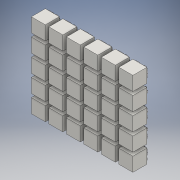
# Autodesk Inventor part: cubes&numbers
Saved by Autodesk Inventor 2017 SP1 (Build 210196100, 196)
## iProperties
Part Number: cubes&numbers
Material: Générique
Document SubType Name: Modeling
Designer: tmonglon
Density: 1 g/cm^3
Appearance: Par défaut
Author: tmonglon
Autodesk Inventor part; units mm, degrees
(part 1 of 3)
ref_plane "YZ Plane" through (0, 0, 0) normal (1, 0, 0) x (0, 1, 0)
ref_plane "XZ Plane" through (0, 0, 0) normal (0, 1, 0) x (-1, 0, 0)
ref_plane "XY Plane" through (0, 0, 0) normal (0, 0, 1) x (1, 0, 0)
sketch "Esquisse1" plane through (0, 0, 0) normal (0, 0, 1) x (1, 0, 0)
  line L0 (0, 0) -> (-8, 0)
  line L1 (-8, 0) -> (-8, 8)
  line L2 (-8, 8) -> (0, 8)
  line L3 (0, 8) -> (0, 0)
  dimension "d0" = 8
  dimension "d1" = 8
  constraints: 8 end point, 2 parallel, 1 horizontal, 1 perpendicular
  measures "d0" distance of L0.start L0.end
  measures "d1" distance of L0.end L1.end
extrude "cube" add sketch "Esquisse1" along normal blind 8
pattern_linear "Réseau rectangulaire1" count 6 spacing 10 along (1, 0, 0) count 5 spacing 10 along (0, 0, 1) of "cube"
sketch "Esquisse5" plane through (-8, 8, 40) normal (0, 1, 0) x (1, 0, 0)
  line L0 (1.5, 39) -> (6.5, 39) construction
  line L1 (6.5, 39) -> (6.5, 33) construction
  line L2 (6.5, 33) -> (1.5, 33) construction
  line L3 (1.5, 33) -> (1.5, 39) construction
  line L4 (0, 40) -> (8, 40) projected
  line L5 (0, 40) -> (0, 32) projected
  line L6 (11.5, 39) -> (16.5, 39) construction
  line L7 (16.5, 39) -> (16.5, 33) construction
  line L8 (16.5, 33) -> (11.5, 33) construction
  line L9 (11.5, 33) -> (11.5, 39) construction
  line L10 (10, 40) -> (18, 40) projected
  line L11 (10, 40) -> (10, 32) projected
  line L12 (21.5, 39) -> (26.5, 39) construction
  line L13 (26.5, 39) -> (26.5, 33) construction
  line L14 (26.5, 33) -> (21.5, 33) construction
  line L15 (21.5, 33) -> (21.5, 39) construction
  line L16 (20, 40) -> (28, 40) projected
  line L17 (20, 40) -> (20, 32) projected
  line L18 (31.5, 39) -> (36.5, 39) construction
  line L19 (36.5, 39) -> (36.5, 33) construction
  line L20 (36.5, 33) -> (31.5, 33) construction
  line L21 (31.5, 33) -> (31.5, 39) construction
  line L22 (30, 40) -> (38, 40) projected
  line L23 (30, 40) -> (30, 32) projected
  line L24 (41.5, 39) -> (46.5, 39) construction
  line L25 (46.5, 39) -> (46.5, 33) construction
  line L26 (46.5, 33) -> (41.5, 33) construction
  line L27 (41.5, 33) -> (41.5, 39) construction
  line L28 (40, 40) -> (48, 40) projected
  line L29 (40, 40) -> (40, 32) projected
  line L30 (51.5, 39) -> (56.5, 39) construction
  line L31 (56.5, 39) -> (56.5, 33) construction
  line L32 (56.5, 33) -> (51.5, 33) construction
  line L33 (51.5, 33) -> (51.5, 39) construction
  line L34 (50, 40) -> (58, 40) projected
  line L35 (50, 40) -> (50, 32) projected
  line L36 (1.5, 29) -> (6.5, 29) construction
  line L37 (6.5, 29) -> (6.5, 23) construction
  line L38 (6.5, 23) -> (1.5, 23) construction
  line L39 (1.5, 23) -> (1.5, 29) construction
  line L40 (0, 30) -> (8, 30) projected
  line L41 (0, 30) -> (0, 22) projected
  line L42 (11.5, 29) -> (16.5, 29) construction
  line L43 (16.5, 29) -> (16.5, 23) construction
  line L44 (16.5, 23) -> (11.5, 23) construction
  line L45 (11.5, 23) -> (11.5, 29) construction
  line L46 (10, 30) -> (18, 30) projected
  line L47 (10, 30) -> (10, 22) projected
  line L48 (21.5, 29) -> (26.5, 29) construction
  line L49 (26.5, 29) -> (26.5, 23) construction
  line L50 (26.5, 23) -> (21.5, 23) construction
  line L51 (21.5, 23) -> (21.5, 29) construction
  line L52 (20, 30) -> (28, 30) projected
  line L53 (20, 30) -> (20, 22) projected
  line L54 (30.5, 29) -> (37.5, 29) construction
  line L55 (37.5, 29) -> (37.5, 23) construction
  line L56 (37.5, 23) -> (30.5, 23) construction
  line L57 (30.5, 23) -> (30.5, 29) construction
  line L58 (30, 30) -> (38, 30) projected
  line L59 (30, 30) -> (30, 22) projected
  line L60 (40.5, 29) -> (47.5, 29) construction
  line L61 (47.5, 29) -> (47.5, 23) construction
  line L62 (47.5, 23) -> (40.5, 23) construction
  line L63 (40.5, 23) -> (40.5, 29) construction
  line L64 (40, 30) -> (48, 30) projected
  line L65 (40, 30) -> (40, 22) projected
  line L66 (50.5, 29) -> (57.5, 29) construction
  line L67 (57.5, 29) -> (57.5, 23) construction
  line L68 (57.5, 23) -> (50.5, 23) construction
  line L69 (50.5, 23) -> (50.5, 29) construction
  line L70 (50, 30) -> (58, 30) projected
  line L71 (50, 30) -> (50, 22) projected
  line L72 (0.5, 19) -> (7.5, 19) construction
  line L73 (7.5, 19) -> (7.5, 13) construction
  line L74 (7.5, 13) -> (0.5, 13) construction
  line L75 (0.5, 13) -> (0.5, 19) construction
  line L76 (0, 20) -> (0, 12) projected
  line L77 (0, 20) -> (8, 20) projected
  line L78 (10.5, 19) -> (17.5, 19) construction
  line L79 (17.5, 19) -> (17.5, 13) construction
  line L80 (17.5, 13) -> (10.5, 13) construction
  line L81 (10.5, 13) -> (10.5, 19) construction
  line L82 (10, 20) -> (18, 20) projected
  line L83 (18, 20) -> (18, 12) projected
  line L84 (20.5, 19) -> (27.5, 19) construction
  line L85 (27.5, 19) -> (27.5, 13) construction
  line L86 (27.5, 13) -> (20.5, 13) construction
  line L87 (20.5, 13) -> (20.5, 19) construction
  line L88 (20, 20) -> (28, 20) projected
  line L89 (28, 20) -> (28, 12) projected
  line L90 (30.5, 19) -> (37.5, 19) construction
  line L91 (37.5, 19) -> (37.5, 13) construction
  line L92 (37.5, 13) -> (30.5, 13) construction
  line L93 (30.5, 13) -> (30.5, 19) construction
  line L94 (30, 20) -> (38, 20) projected
  line L95 (30, 20) -> (30, 12) projected
  line L96 (40.5, 19) -> (47.5, 19) construction
  line L97 (47.5, 19) -> (47.5, 13) construction
  line L98 (47.5, 13) -> (40.5, 13) construction
  line L99 (40.5, 13) -> (40.5, 19) construction
  line L100 (40, 20) -> (48, 20) projected
  line L101 (40, 20) -> (40, 12) projected
  line L102 (50.5, 19) -> (57.5, 19) construction
  line L103 (57.5, 19) -> (57.5, 13) construction
  line L104 (57.5, 13) -> (50.5, 13) construction
  line L105 (50.5, 13) -> (50.5, 19) construction
  line L106 (50, 20) -> (58, 20) projected
  line L107 (58, 20) -> (58, 12) projected
  line L108 (0.5, 9) -> (7.5, 9) construction
  line L109 (7.5, 9) -> (7.5, 3) construction
  line L110 (7.5, 3) -> (0.5, 3) construction
  line L111 (0.5, 3) -> (0.5, 9) construction
  line L112 (0, 10) -> (8, 10) projected
  line L113 (8, 10) -> (8, 2) projected
  line L114 (10.5, 9) -> (17.5, 9) construction
  line L115 (17.5, 9) -> (17.5, 3) construction
  line L116 (17.5, 3) -> (10.5, 3) construction
  line L117 (10.5, 3) -> (10.5, 9) construction
  line L118 (10, 10) -> (18, 10) projected
  line L119 (18, 10) -> (18, 2) projected
  line L120 (20.5, 9) -> (27.5, 9) construction
  line L121 (27.5, 9) -> (27.5, 3) construction
  line L122 (27.5, 3) -> (20.5, 3) construction
  line L123 (20.5, 3) -> (20.5, 9) construction
  line L124 (20, 10) -> (28, 10) projected
  line L125 (28, 10) -> (28, 2) projected
  line L126 (30.5, 9) -> (37.5, 9) construction
  line L127 (37.5, 9) -> (37.5, 3) construction
  line L128 (37.5, 3) -> (30.5, 3) construction
  line L129 (30.5, 3) -> (30.5, 9) construction
  line L130 (30, 10) -> (38, 10) projected
  line L131 (38, 10) -> (38, 2) projected
  line L132 (40.5, 9) -> (47.5, 9) construction
  line L133 (47.5, 9) -> (47.5, 3) construction
  line L134 (47.5, 3) -> (40.5, 3) construction
  line L135 (40.5, 3) -> (40.5, 9) construction
  line L136 (40, 10) -> (48, 10) projected
  line L137 (48, 10) -> (48, 2) projected
  line L138 (50.5, 9) -> (57.5, 9) construction
  line L139 (57.5, 9) -> (57.5, 3) construction
  line L140 (57.5, 3) -> (50.5, 3) construction
  line L141 (50.5, 3) -> (50.5, 9) construction
  line L142 (50, 10) -> (58, 10) projected
  line L143 (50, 10) -> (50, 2) projected
  line L144 (0.5, -1) -> (7.5, -1) construction
  line L145 (7.5, -1) -> (7.5, -7) construction
  line L146 (7.5, -7) -> (0.5, -7) construction
  line L147 (0.5, -7) -> (0.5, -1) construction
  line L148 (0, 0) -> (8, 0) projected
  line L149 (0, 0) -> (0, -8) projected
  line L150 (10.5, -1) -> (17.5, -1) construction
  line L151 (17.5, -1) -> (17.5, -7) construction
  line L152 (17.5, -7) -> (10.5, -7) construction
  line L153 (10.5, -7) -> (10.5, -1) construction
  line L154 (10, 0) -> (18, 0) projected
  line L155 (18, 0) -> (18, -8) projected
  line L156 (20.5, -1) -> (27.5, -1) construction
  line L157 (27.5, -1) -> (27.5, -7) construction
  line L158 (27.5, -7) -> (20.5, -7) construction
  line L159 (20.5, -7) -> (20.5, -1) construction
  line L160 (20, 0) -> (28, 0) projected
  line L161 (20, 0) -> (20, -8) projected
  line L162 (30.5, -1) -> (37.5, -1) construction
  line L163 (37.5, -1) -> (37.5, -7) construction
  line L164 (37.5, -7) -> (30.5, -7) construction
  line L165 (30.5, -7) -> (30.5, -1) construction
  line L166 (30, 0) -> (38, 0) projected
  line L167 (30, 0) -> (30, -8) projected
  line L168 (40.5, -1) -> (47.5, -1) construction
  line L169 (47.5, -1) -> (47.5, -7) construction
  line L170 (47.5, -7) -> (40.5, -7) construction
  line L171 (40.5, -7) -> (40.5, -1) construction
  line L172 (40, 0) -> (48, 0) projected
  line L173 (48, 0) -> (48, -8) projected
  line L174 (50.5, -1) -> (57.5, -1) construction
  line L175 (57.5, -1) -> (57.5, -7) construction
  line L176 (57.5, -7) -> (50.5, -7) construction
  line L177 (50.5, -7) -> (50.5, -1) construction
  line L178 (50, 0) -> (58, 0) projected
  line L179 (50, 0) -> (50, -8) projected
  spline S0 degree 2 poles (3.7776, 35.8264) (3.7776, 35.0355) (3.5996, 33.8491) (3.4068, 33.4487) knots 0 0 0 1 2 2 2
  spline S1 degree 2 poles (3.4068, 33.4487) (3.2091, 33.0532) (2.5862, 32.6479) (2.1364, 32.6479) knots 0 0 0 1 2 2 2
  spline S2 degree 2 poles (2.1364, 32.6479) (1.6865, 32.6479) (1.0588, 33.0532) (0.861, 33.4586) knots 0 0 0 1 2 2 2
  spline S3 degree 2 poles (0.861, 33.4586) (0.6682, 33.859) (0.4903, 35.0355) (0.4903, 35.8264) knots 0 0 0 1 2 2 2
  spline S4 degree 2 poles (0.4903, 35.8264) (0.4903, 36.6371) (0.6633, 37.784) (0.866, 38.1992) knots 0 0 0 1 2 2 2
  spline S5 degree 2 poles (0.866, 38.1992) (1.0686, 38.6045) (1.6964, 39) (2.1364, 39) knots 0 0 0 1 2 2 2
  spline S6 degree 2 poles (2.1364, 39) (2.5961, 39) (3.2091, 38.5848) (3.4068, 38.1745) knots 0 0 0 1 2 2 2
  spline S7 degree 2 poles (3.4068, 38.1745) (3.6045, 37.7741) (3.7776, 36.5926) (3.7776, 35.8264) knots 0 0 0 1 2 2 2
  spline S8 degree 2 poles (2.7049, 35.8264) (2.7049, 36.9584) (2.4429, 37.8729) (2.1364, 37.8729) knots 0 0 0 1 2 2 2
  spline S9 degree 2 poles (2.1364, 37.8729) (1.825, 37.8729) (1.563, 36.9584) (1.563, 35.8215) knots 0 0 0 1 2 2 2
  spline S10 degree 2 poles (1.563, 35.8215) (1.563, 34.7043) (1.825, 33.775) (2.1364, 33.775) knots 0 0 0 1 2 2 2
  spline S11 degree 2 poles (2.1364, 33.775) (2.4429, 33.775) (2.7049, 34.7043) (2.7049, 35.8264) knots 0 0 0 1 2 2 2
  line L180 (7.3763, 32.7764) -> (4.5586, 32.7764)
  line L181 (4.5586, 32.7764) -> (4.5586, 33.8392)
  line L182 (4.5586, 33.8392) -> (5.4583, 33.8392)
  line L183 (5.4583, 33.8392) -> (5.4583, 37.0672)
  line L184 (5.4583, 37.0672) -> (4.5586, 37.0672)
  line L185 (4.5586, 37.0672) -> (4.5586, 38.0608)
  spline S12 degree 2 poles (4.5586, 38.0608) (4.7563, 38.0608) (5.1468, 38.1349) (5.2655, 38.214) knots 0 0 0 1 2 2 2
  spline S13 degree 2 poles (5.2655, 38.214) (5.3989, 38.3129) (5.5522, 38.6441) (5.5621, 38.8912) knots 0 0 0 1 2 2 2
  line L186 (5.5621, 38.8912) -> (6.4964, 38.8912)
  line L187 (6.4964, 38.8912) -> (6.4964, 33.8392)
  line L188 (6.4964, 33.8392) -> (7.3763, 33.8392)
  line L189 (7.3763, 33.8392) -> (7.3763, 32.7764)
  spline S14 degree 2 poles (13.7776, 35.8264) (13.7776, 35.0355) (13.5996, 33.8491) (13.4068, 33.4487) knots 0 0 0 1 2 2 2
  spline S15 degree 2 poles (13.4068, 33.4487) (13.2091, 33.0532) (12.5862, 32.6479) (12.1364, 32.6479) knots 0 0 0 1 2 2 2
  spline S16 degree 2 poles (12.1364, 32.6479) (11.6865, 32.6479) (11.0588, 33.0532) (10.861, 33.4586) knots 0 0 0 1 2 2 2
  spline S17 degree 2 poles (10.861, 33.4586) (10.6682, 33.859) (10.4903, 35.0355) (10.4903, 35.8264) knots 0 0 0 1 2 2 2
  spline S18 degree 2 poles (10.4903, 35.8264) (10.4903, 36.6371) (10.6633, 37.784) (10.866, 38.1992) knots 0 0 0 1 2 2 2
  spline S19 degree 2 poles (10.866, 38.1992) (11.0686, 38.6045) (11.6964, 39) (12.1364, 39) knots 0 0 0 1 2 2 2
  spline S20 degree 2 poles (12.1364, 39) (12.5961, 39) (13.2091, 38.5848) (13.4068, 38.1745) knots 0 0 0 1 2 2 2
  spline S21 degree 2 poles (13.4068, 38.1745) (13.6045, 37.7741) (13.7776, 36.5926) (13.7776, 35.8264) knots 0 0 0 1 2 2 2
  spline S22 degree 2 poles (12.7049, 35.8264) (12.7049, 36.9584) (12.4429, 37.8729) (12.1364, 37.8729) knots 0 0 0 1 2 2 2
  spline S23 degree 2 poles (12.1364, 37.8729) (11.825, 37.8729) (11.563, 36.9584) (11.563, 35.8215) knots 0 0 0 1 2 2 2
  spline S24 degree 2 poles (11.563, 35.8215) (11.563, 34.7043) (11.825, 33.775) (12.1364, 33.775) knots 0 0 0 1 2 2 2
  spline S25 degree 2 poles (12.1364, 33.775) (12.4429, 33.775) (12.7049, 34.7043) (12.7049, 35.8264) knots 0 0 0 1 2 2 2
  line L190 (17.5641, 32.7764) -> (14.4301, 32.7764)
  line L191 (14.4301, 32.7764) -> (14.4301, 33.77)
  spline S26 degree 2 poles (14.4301, 33.77) (14.8305, 34.2248) (15.4583, 35.0256) (15.7005, 35.3865) knots 0 0 0 1 2 2 2
  spline S27 degree 2 poles (15.7005, 35.3865) (16.0119, 35.8561) (16.2937, 36.5729) (16.2937, 36.9485) knots 0 0 0 1 2 2 2
  spline S28 degree 2 poles (16.2937, 36.9485) (16.2937, 37.3737) (15.9378, 37.8284) (15.6214, 37.8284) knots 0 0 0 1 2 2 2
  spline S29 degree 2 poles (15.6214, 37.8284) (15.4583, 37.8284) (15.1716, 37.7147) (15.0183, 37.6258) knots 0 0 0 1 2 2 2
  spline S30 degree 2 poles (15.0183, 37.6258) (14.875, 37.5318) (14.6673, 37.3341) (14.6179, 37.2847) knots 0 0 0 1 2 2 2
  line L192 (14.6179, 37.2847) -> (14.5339, 37.2847)
  line L193 (14.5339, 37.2847) -> (14.5339, 38.6144)
  spline S31 degree 2 poles (14.5339, 38.6144) (14.7118, 38.738) (15.483, 38.9951) (15.834, 38.9951) knots 0 0 0 1 2 2 2
  spline S32 degree 2 poles (15.834, 38.9951) (16.5952, 38.9951) (17.3763, 38.0262) (17.3763, 37.1512) knots 0 0 0 1 2 2 2
  spline S33 degree 2 poles (17.3763, 37.1512) (17.3763, 36.6124) (17.0203, 35.5743) (16.61, 34.9811) knots 0 0 0 1 2 2 2
  spline S34 degree 2 poles (16.61, 34.9811) (16.353, 34.6153) (15.8636, 34.0468) (15.7549, 33.9282) knots 0 0 0 1 2 2 2
  line L194 (15.7549, 33.9282) -> (17.5641, 33.9282)
  line L195 (17.5641, 33.9282) -> (17.5641, 32.7764)
  spline S35 degree 2 poles (23.7776, 35.8215) (23.7776, 35.0306) (23.5996, 33.8442) (23.4068, 33.4438) knots 0 0 0 1 2 2 2
  spline S36 degree 2 poles (23.4068, 33.4438) (23.2091, 33.0483) (22.5862, 32.6429) (22.1364, 32.6429) knots 0 0 0 1 2 2 2
  spline S37 degree 2 poles (22.1364, 32.6429) (21.6865, 32.6429) (21.0588, 33.0483) (20.861, 33.4536) knots 0 0 0 1 2 2 2
  spline S38 degree 2 poles (20.861, 33.4536) (20.6682, 33.8541) (20.4903, 35.0306) (20.4903, 35.8215) knots 0 0 0 1 2 2 2
  spline S39 degree 2 poles (20.4903, 35.8215) (20.4903, 36.6322) (20.6633, 37.779) (20.866, 38.1942) knots 0 0 0 1 2 2 2
  spline S40 degree 2 poles (20.866, 38.1942) (21.0686, 38.5996) (21.6964, 38.9951) (22.1364, 38.9951) knots 0 0 0 1 2 2 2
  spline S41 degree 2 poles (22.1364, 38.9951) (22.5961, 38.9951) (23.2091, 38.5798) (23.4068, 38.1695) knots 0 0 0 1 2 2 2
  spline S42 degree 2 poles (23.4068, 38.1695) (23.6045, 37.7691) (23.7776, 36.5877) (23.7776, 35.8215) knots 0 0 0 1 2 2 2
  spline S43 degree 2 poles (22.7049, 35.8215) (22.7049, 36.9535) (22.4429, 37.868) (22.1364, 37.868) knots 0 0 0 1 2 2 2
  spline S44 degree 2 poles (22.1364, 37.868) (21.825, 37.868) (21.563, 36.9535) (21.563, 35.8165) knots 0 0 0 1 2 2 2
  spline S45 degree 2 poles (21.563, 35.8165) (21.563, 34.6994) (21.825, 33.77) (22.1364, 33.77) knots 0 0 0 1 2 2 2
  spline S46 degree 2 poles (22.1364, 33.77) (22.4429, 33.77) (22.7049, 34.6994) (22.7049, 35.8215) knots 0 0 0 1 2 2 2
  spline S47 degree 2 poles (27.4553, 34.6203) (27.4553, 34.1704) (27.223, 33.4339) (27.0006, 33.1768) knots 0 0 0 1 2 2 2
  spline S48 degree 2 poles (27.0006, 33.1768) (26.7732, 32.9198) (26.1652, 32.6429) (25.7301, 32.6429) knots 0 0 0 1 2 2 2
  spline S49 degree 2 poles (25.7301, 32.6429) (25.2309, 32.6429) (24.519, 32.8802) (24.2966, 33.0285) knots 0 0 0 1 2 2 2
  line L196 (24.2966, 33.0285) -> (24.2966, 34.3533)
  line L197 (24.2966, 34.3533) -> (24.4004, 34.3533)
  spline S50 degree 2 poles (24.4004, 34.3533) (24.6327, 34.1408) (25.2655, 33.8244) (25.5275, 33.8244) knots 0 0 0 1 2 2 2
  spline S51 degree 2 poles (25.5275, 33.8244) (25.6807, 33.8244) (26.0465, 33.9035) (26.1701, 34.032) knots 0 0 0 1 2 2 2
  spline S52 degree 2 poles (26.1701, 34.032) (26.264, 34.1358) (26.3827, 34.4374) (26.3827, 34.7092) knots 0 0 0 1 2 2 2
  spline S53 degree 2 poles (26.3827, 34.7092) (26.3827, 34.9811) (26.2146, 35.2728) (26.0811, 35.342) knots 0 0 0 1 2 2 2
  spline S54 degree 2 poles (26.0811, 35.342) (25.9427, 35.4112) (25.5571, 35.426) (25.4138, 35.426) knots 0 0 0 1 2 2 2
  line L198 (25.4138, 35.426) -> (25.2309, 35.426)
  line L199 (25.2309, 35.426) -> (25.2309, 36.4987)
  line L200 (25.2309, 36.4987) -> (25.3989, 36.4987)
  spline S55 degree 2 poles (25.3989, 36.4987) (25.5917, 36.4987) (25.913, 36.5481) (26.0267, 36.6223) knots 0 0 0 1 2 2 2
  spline S56 degree 2 poles (26.0267, 36.6223) (26.1404, 36.7014) (26.269, 36.9782) (26.269, 37.2155) knots 0 0 0 1 2 2 2
  spline S57 degree 2 poles (26.269, 37.2155) (26.269, 37.4033) (26.1503, 37.6357) (26.0613, 37.6999) knots 0 0 0 1 2 2 2
  spline S58 degree 2 poles (26.0613, 37.6999) (25.9575, 37.7741) (25.6857, 37.8235) (25.5868, 37.8235) knots 0 0 0 1 2 2 2
  spline S59 degree 2 poles (25.5868, 37.8235) (25.4335, 37.8235) (25.1073, 37.7197) (24.9541, 37.6357) knots 0 0 0 1 2 2 2
  spline S60 degree 2 poles (24.9541, 37.6357) (24.8354, 37.5714) (24.5734, 37.3638) (24.5092, 37.3094) knots 0 0 0 1 2 2 2
  line L201 (24.5092, 37.3094) -> (24.4202, 37.3094)
  line L202 (24.4202, 37.3094) -> (24.4202, 38.6144)
  spline S61 degree 2 poles (24.4202, 38.6144) (24.6377, 38.7479) (25.3841, 39) (25.7746, 39) knots 0 0 0 1 2 2 2
  spline S62 degree 2 poles (25.7746, 39) (26.1553, 39) (26.7089, 38.8122) (26.9066, 38.6293) knots 0 0 0 1 2 2 2
  spline S63 degree 2 poles (26.9066, 38.6293) (27.1241, 38.4365) (27.3417, 37.8433) (27.3417, 37.4725) knots 0 0 0 1 2 2 2
  spline S64 degree 2 poles (27.3417, 37.4725) (27.3417, 36.9485) (26.9215, 36.1675) (26.5804, 36.0538) knots 0 0 0 1 2 2 2
  line L203 (26.5804, 36.0538) -> (26.5804, 35.9945)
  spline S65 degree 2 poles (26.5804, 35.9945) (26.7336, 35.9648) (27.0203, 35.8066) (27.1588, 35.6287) knots 0 0 0 1 2 2 2
  spline S66 degree 2 poles (27.1588, 35.6287) (27.2873, 35.4705) (27.4553, 34.9663) (27.4553, 34.6203) knots 0 0 0 1 2 2 2
  spline S67 degree 2 poles (33.7776, 35.8264) (33.7776, 35.0355) (33.5996, 33.8491) (33.4068, 33.4487) knots 0 0 0 1 2 2 2
  spline S68 degree 2 poles (33.4068, 33.4487) (33.2091, 33.0532) (32.5862, 32.6479) (32.1364, 32.6479) knots 0 0 0 1 2 2 2
  spline S69 degree 2 poles (32.1364, 32.6479) (31.6865, 32.6479) (31.0588, 33.0532) (30.861, 33.4586) knots 0 0 0 1 2 2 2
  spline S70 degree 2 poles (30.861, 33.4586) (30.6682, 33.859) (30.4903, 35.0355) (30.4903, 35.8264) knots 0 0 0 1 2 2 2
  spline S71 degree 2 poles (30.4903, 35.8264) (30.4903, 36.6371) (30.6633, 37.784) (30.866, 38.1992) knots 0 0 0 1 2 2 2
  spline S72 degree 2 poles (30.866, 38.1992) (31.0686, 38.6045) (31.6964, 39) (32.1364, 39) knots 0 0 0 1 2 2 2
  spline S73 degree 2 poles (32.1364, 39) (32.5961, 39) (33.2091, 38.5848) (33.4068, 38.1745) knots 0 0 0 1 2 2 2
  spline S74 degree 2 poles (33.4068, 38.1745) (33.6045, 37.7741) (33.7776, 36.5926) (33.7776, 35.8264) knots 0 0 0 1 2 2 2
  spline S75 degree 2 poles (32.7049, 35.8264) (32.7049, 36.9584) (32.4429, 37.8729) (32.1364, 37.8729) knots 0 0 0 1 2 2 2
  spline S76 degree 2 poles (32.1364, 37.8729) (31.825, 37.8729) (31.563, 36.9584) (31.563, 35.8215) knots 0 0 0 1 2 2 2
  spline S77 degree 2 poles (31.563, 35.8215) (31.563, 34.7043) (31.825, 33.775) (32.1364, 33.775) knots 0 0 0 1 2 2 2
  spline S78 degree 2 poles (32.1364, 33.775) (32.4429, 33.775) (32.7049, 34.7043) (32.7049, 35.8264) knots 0 0 0 1 2 2 2
  line L204 (37.6086, 34.2001) -> (37.0352, 34.2001)
  line L205 (37.0352, 34.2001) -> (37.0352, 32.7616)
  line L206 (37.0352, 32.7616) -> (35.9971, 32.7616)
  line L207 (35.9971, 32.7616) -> (35.9971, 34.2001)
  line L208 (35.9971, 34.2001) -> (34.1285, 34.2001)
  line L209 (34.1285, 34.2001) -> (34.1285, 35.337)
  line L210 (34.1285, 35.337) -> (35.9625, 38.8764)
  line L211 (35.9625, 38.8764) -> (37.0352, 38.8764)
  line L212 (37.0352, 38.8764) -> (37.0352, 35.2975)
  line L213 (37.0352, 35.2975) -> (37.6086, 35.2975)
  line L214 (37.6086, 35.2975) -> (37.6086, 34.2001)
  line L215 (35.9971, 35.2975) -> (35.9971, 37.3687)
  line L216 (35.9971, 37.3687) -> (34.9244, 35.2975)
  line L217 (34.9244, 35.2975) -> (35.9971, 35.2975)
  spline S79 degree 2 poles (43.7776, 35.8264) (43.7776, 35.0355) (43.5996, 33.8491) (43.4068, 33.4487) knots 0 0 0 1 2 2 2
  spline S80 degree 2 poles (43.4068, 33.4487) (43.2091, 33.0532) (42.5862, 32.6479) (42.1364, 32.6479) knots 0 0 0 1 2 2 2
  spline S81 degree 2 poles (42.1364, 32.6479) (41.6865, 32.6479) (41.0588, 33.0532) (40.861, 33.4586) knots 0 0 0 1 2 2 2
  spline S82 degree 2 poles (40.861, 33.4586) (40.6682, 33.859) (40.4903, 35.0355) (40.4903, 35.8264) knots 0 0 0 1 2 2 2
  spline S83 degree 2 poles (40.4903, 35.8264) (40.4903, 36.6371) (40.6633, 37.784) (40.866, 38.1992) knots 0 0 0 1 2 2 2
  spline S84 degree 2 poles (40.866, 38.1992) (41.0686, 38.6045) (41.6964, 39) (42.1364, 39) knots 0 0 0 1 2 2 2
  spline S85 degree 2 poles (42.1364, 39) (42.5961, 39) (43.2091, 38.5848) (43.4068, 38.1745) knots 0 0 0 1 2 2 2
  spline S86 degree 2 poles (43.4068, 38.1745) (43.6045, 37.7741) (43.7776, 36.5926) (43.7776, 35.8264) knots 0 0 0 1 2 2 2
  spline S87 degree 2 poles (42.7049, 35.8264) (42.7049, 36.9584) (42.4429, 37.8729) (42.1364, 37.8729) knots 0 0 0 1 2 2 2
  spline S88 degree 2 poles (42.1364, 37.8729) (41.825, 37.8729) (41.563, 36.9584) (41.563, 35.8215) knots 0 0 0 1 2 2 2
  spline S89 degree 2 poles (41.563, 35.8215) (41.563, 34.7043) (41.825, 33.775) (42.1364, 33.775) knots 0 0 0 1 2 2 2
  spline S90 degree 2 poles (42.1364, 33.775) (42.4429, 33.775) (42.7049, 34.7043) (42.7049, 35.8264) knots 0 0 0 1 2 2 2
  spline S91 degree 2 poles (47.4652, 34.8427) (47.4652, 34.3632) (47.2378, 33.5525) (47.0154, 33.2609) knots 0 0 0 1 2 2 2
  spline S92 degree 2 poles (47.0154, 33.2609) (46.7929, 32.9692) (46.175, 32.6479) (45.7252, 32.6479) knots 0 0 0 1 2 2 2
  spline S93 degree 2 poles (45.7252, 32.6479) (45.2506, 32.6528) (44.5685, 32.8753) (44.346, 33.0186) knots 0 0 0 1 2 2 2
  line L218 (44.346, 33.0186) -> (44.346, 34.3484)
  line L219 (44.346, 34.3484) -> (44.4449, 34.3484)
  spline S94 degree 2 poles (44.4449, 34.3484) (44.524, 34.2841) (44.7217, 34.116) (44.8848, 34.0271) knots 0 0 0 1 2 2 2
  spline S95 degree 2 poles (44.8848, 34.0271) (45.0381, 33.943) (45.3495, 33.8293) (45.5423, 33.8293) knots 0 0 0 1 2 2 2
  spline S96 degree 2 poles (45.5423, 33.8293) (45.7104, 33.8293) (46.091, 33.948) (46.2096, 34.1062) knots 0 0 0 1 2 2 2
  spline S97 degree 2 poles (46.2096, 34.1062) (46.2937, 34.2297) (46.3925, 34.5313) (46.3925, 34.7834) knots 0 0 0 1 2 2 2
  spline S98 degree 2 poles (46.3925, 34.7834) (46.3925, 35.0009) (46.269, 35.3074) (46.1701, 35.4013) knots 0 0 0 1 2 2 2
  spline S99 degree 2 poles (46.1701, 35.4013) (46.0218, 35.5397) (45.6115, 35.6188) (45.4632, 35.6188) knots 0 0 0 1 2 2 2
  spline S100 degree 2 poles (45.4632, 35.6188) (45.2259, 35.6188) (44.786, 35.51) (44.6229, 35.4507) knots 0 0 0 1 2 2 2
  line L220 (44.6229, 35.4507) -> (44.5289, 35.4507)
  line L221 (44.5289, 35.4507) -> (44.5289, 38.8764)
  line L222 (44.5289, 38.8764) -> (47.3466, 38.8764)
  line L223 (47.3466, 38.8764) -> (47.3466, 37.7246)
  line L224 (47.3466, 37.7246) -> (45.5374, 37.7246)
  line L225 (45.5374, 37.7246) -> (45.5374, 36.7113)
  spline S101 degree 2 poles (45.5374, 36.7113) (45.6214, 36.7212) (45.8587, 36.731) (45.9279, 36.731) knots 0 0 0 1 2 2 2
  spline S102 degree 2 poles (45.9279, 36.731) (46.2344, 36.731) (46.7534, 36.5531) (46.9511, 36.3702) knots 0 0 0 1 2 2 2
  spline S103 degree 2 poles (46.9511, 36.3702) (47.1983, 36.1428) (47.4652, 35.3865) (47.4652, 34.8427) knots 0 0 0 1 2 2 2
  spline S104 degree 2 poles (53.7776, 35.8264) (53.7776, 35.0355) (53.5996, 33.8491) (53.4068, 33.4487) knots 0 0 0 1 2 2 2
  spline S105 degree 2 poles (53.4068, 33.4487) (53.2091, 33.0532) (52.5862, 32.6479) (52.1364, 32.6479) knots 0 0 0 1 2 2 2
  spline S106 degree 2 poles (52.1364, 32.6479) (51.6865, 32.6479) (51.0588, 33.0532) (50.861, 33.4586) knots 0 0 0 1 2 2 2
  spline S107 degree 2 poles (50.861, 33.4586) (50.6682, 33.859) (50.4903, 35.0355) (50.4903, 35.8264) knots 0 0 0 1 2 2 2
  spline S108 degree 2 poles (50.4903, 35.8264) (50.4903, 36.6371) (50.6633, 37.784) (50.866, 38.1992) knots 0 0 0 1 2 2 2
  spline S109 degree 2 poles (50.866, 38.1992) (51.0686, 38.6045) (51.6964, 39) (52.1364, 39) knots 0 0 0 1 2 2 2
  spline S110 degree 2 poles (52.1364, 39) (52.5961, 39) (53.2091, 38.5848) (53.4068, 38.1745) knots 0 0 0 1 2 2 2
  spline S111 degree 2 poles (53.4068, 38.1745) (53.6045, 37.7741) (53.7776, 36.5926) (53.7776, 35.8264) knots 0 0 0 1 2 2 2
  spline S112 degree 2 poles (52.7049, 35.8264) (52.7049, 36.9584) (52.4429, 37.8729) (52.1364, 37.8729) knots 0 0 0 1 2 2 2
  spline S113 degree 2 poles (52.1364, 37.8729) (51.825, 37.8729) (51.563, 36.9584) (51.563, 35.8215) knots 0 0 0 1 2 2 2
  spline S114 degree 2 poles (51.563, 35.8215) (51.563, 34.7043) (51.825, 33.775) (52.1364, 33.775) knots 0 0 0 1 2 2 2
  spline S115 degree 2 poles (52.1364, 33.775) (52.4429, 33.775) (52.7049, 34.7043) (52.7049, 35.8264) knots 0 0 0 1 2 2 2
  spline S116 degree 2 poles (57.5394, 34.8526) (57.5394, 33.8887) (56.6842, 32.6479) (55.9427, 32.6479) knots 0 0 0 1 2 2 2
  spline S117 degree 2 poles (55.9427, 32.6479) (55.572, 32.6479) (54.9837, 32.9544) (54.781, 33.2559) knots 0 0 0 1 2 2 2
  spline S118 degree 2 poles (54.781, 33.2559) (54.5388, 33.6069) (54.2818, 34.7191) (54.2818, 35.4952) knots 0 0 0 1 2 2 2
  spline S119 degree 2 poles (54.2818, 35.4952) (54.2818, 36.296) (54.524, 37.5417) (54.7959, 38.0212) knots 0 0 0 1 2 2 2
  spline S120 degree 2 poles (54.7959, 38.0212) (55.0529, 38.476) (55.8982, 38.9901) (56.4716, 38.9901) knots 0 0 0 1 2 2 2
  spline S121 degree 2 poles (56.4716, 38.9901) (56.6793, 38.9901) (57.0994, 38.911) (57.1785, 38.8863) knots 0 0 0 1 2 2 2
  line L226 (57.1785, 38.8863) -> (57.1785, 37.69)
  line L227 (57.1785, 37.69) -> (57.0994, 37.69)
  spline S122 degree 2 poles (57.0994, 37.69) (57.0253, 37.7444) (56.6842, 37.8779) (56.4618, 37.8779) knots 0 0 0 1 2 2 2
  spline S123 degree 2 poles (56.4618, 37.8779) (55.9625, 37.8779) (55.4187, 37.1216) (55.3545, 36.4196) knots 0 0 0 1 2 2 2
  spline S124 degree 2 poles (55.3545, 36.4196) (55.567, 36.6124) (55.9971, 36.8398) (56.269, 36.8398) knots 0 0 0 1 2 2 2
  spline S125 degree 2 poles (56.269, 36.8398) (56.4964, 36.8398) (56.9017, 36.6618) (57.0599, 36.4938) knots 0 0 0 1 2 2 2
  spline S126 degree 2 poles (57.0599, 36.4938) (57.2774, 36.2515) (57.5394, 35.4656) (57.5394, 34.8526) knots 0 0 0 1 2 2 2
  spline S127 degree 2 poles (56.2937, 33.9331) (56.3777, 34.0814) (56.4667, 34.4275) (56.4667, 34.7784) knots 0 0 0 1 2 2 2
  spline S128 degree 2 poles (56.4667, 34.7784) (56.4667, 35.075) (56.3629, 35.4606) (56.269, 35.5743) knots 0 0 0 1 2 2 2
  spline S129 degree 2 poles (56.269, 35.5743) (56.175, 35.6929) (55.9378, 35.777) (55.7994, 35.777) knots 0 0 0 1 2 2 2
  spline S130 degree 2 poles (55.7994, 35.777) (55.6906, 35.777) (55.4533, 35.6929) (55.3495, 35.6336) knots 0 0 0 1 2 2 2
  spline S131 degree 2 poles (55.3495, 35.6336) (55.3495, 35.5941) (55.3446, 35.4062) (55.3446, 35.2629) knots 0 0 0 1 2 2 2
  spline S132 degree 2 poles (55.3446, 35.2629) (55.3446, 34.734) (55.4731, 34.0963) (55.572, 33.9331) knots 0 0 0 1 2 2 2
  spline S133 degree 2 poles (55.572, 33.9331) (55.6461, 33.7997) (55.834, 33.686) (55.9427, 33.686) knots 0 0 0 1 2 2 2
  spline S134 degree 2 poles (55.9427, 33.686) (56.0267, 33.686) (56.2245, 33.8096) (56.2937, 33.9331) knots 0 0 0 1 2 2 2
  spline S135 degree 2 poles (3.7776, 25.8264) (3.7776, 25.0355) (3.5996, 23.8491) (3.4068, 23.4487) knots 0 0 0 1 2 2 2
  spline S136 degree 2 poles (3.4068, 23.4487) (3.2091, 23.0532) (2.5862, 22.6479) (2.1364, 22.6479) knots 0 0 0 1 2 2 2
  spline S137 degree 2 poles (2.1364, 22.6479) (1.6865, 22.6479) (1.0588, 23.0532) (0.861, 23.4586) knots 0 0 0 1 2 2 2
  spline S138 degree 2 poles (0.861, 23.4586) (0.6682, 23.859) (0.4903, 25.0355) (0.4903, 25.8264) knots 0 0 0 1 2 2 2
  spline S139 degree 2 poles (0.4903, 25.8264) (0.4903, 26.6371) (0.6633, 27.784) (0.866, 28.1992) knots 0 0 0 1 2 2 2
  spline S140 degree 2 poles (0.866, 28.1992) (1.0686, 28.6045) (1.6964, 29) (2.1364, 29) knots 0 0 0 1 2 2 2
  spline S141 degree 2 poles (2.1364, 29) (2.5961, 29) (3.2091, 28.5848) (3.4068, 28.1745) knots 0 0 0 1 2 2 2
  spline S142 degree 2 poles (3.4068, 28.1745) (3.6045, 27.7741) (3.7776, 26.5926) (3.7776, 25.8264) knots 0 0 0 1 2 2 2
  spline S143 degree 2 poles (2.7049, 25.8264) (2.7049, 26.9584) (2.4429, 27.8729) (2.1364, 27.8729) knots 0 0 0 1 2 2 2
  spline S144 degree 2 poles (2.1364, 27.8729) (1.825, 27.8729) (1.563, 26.9584) (1.563, 25.8215) knots 0 0 0 1 2 2 2
  spline S145 degree 2 poles (1.563, 25.8215) (1.563, 24.7043) (1.825, 23.775) (2.1364, 23.775) knots 0 0 0 1 2 2 2
  spline S146 degree 2 poles (2.1364, 23.775) (2.4429, 23.775) (2.7049, 24.7043) (2.7049, 25.8264) knots 0 0 0 1 2 2 2
  line L228 (7.4702, 27.6653) -> (5.656, 22.7764)
  line L229 (5.656, 22.7764) -> (4.4647, 22.7764)
  line L230 (4.4647, 22.7764) -> (6.3678, 27.7246)
  line L231 (6.3678, 27.7246) -> (4.3361, 27.7246)
  line L232 (4.3361, 27.7246) -> (4.3361, 28.8764)
  line L233 (4.3361, 28.8764) -> (7.4702, 28.8764)
  line L234 (7.4702, 28.8764) -> (7.4702, 27.6653)
  line L235 (3.6441, 12.7715) -> (0.8264, 12.7715)
  line L236 (0.8264, 12.7715) -> (0.8264, 13.8343)
  line L237 (0.8264, 13.8343) -> (1.7261, 13.8343)
  line L238 (1.7261, 13.8343) -> (1.7261, 17.0622)
  line L239 (1.7261, 17.0622) -> (0.8264, 17.0622)
  line L240 (0.8264, 17.0622) -> (0.8264, 18.0558)
  spline S147 degree 2 poles (0.8264, 18.0558) (1.0241, 18.0558) (1.4147, 18.13) (1.5333, 18.2091) knots 0 0 0 1 2 2 2
  spline S148 degree 2 poles (1.5333, 18.2091) (1.6668, 18.3079) (1.82, 18.6391) (1.8299, 18.8863) knots 0 0 0 1 2 2 2
  line L241 (1.8299, 18.8863) -> (2.7642, 18.8863)
  line L242 (2.7642, 18.8863) -> (2.7642, 13.8343)
  line L243 (2.7642, 13.8343) -> (3.6441, 13.8343)
  line L244 (3.6441, 13.8343) -> (3.6441, 12.7715)
  spline S149 degree 2 poles (7.4553, 14.6203) (7.4553, 14.1704) (7.223, 13.4339) (7.0006, 13.1768) knots 0 0 0 1 2 2 2
  spline S150 degree 2 poles (7.0006, 13.1768) (6.7732, 12.9198) (6.1652, 12.6429) (5.7301, 12.6429) knots 0 0 0 1 2 2 2
  spline S151 degree 2 poles (5.7301, 12.6429) (5.2309, 12.6429) (4.519, 12.8802) (4.2966, 13.0285) knots 0 0 0 1 2 2 2
  line L245 (4.2966, 13.0285) -> (4.2966, 14.3533)
  line L246 (4.2966, 14.3533) -> (4.4004, 14.3533)
  spline S152 degree 2 poles (4.4004, 14.3533) (4.6327, 14.1408) (5.2655, 13.8244) (5.5275, 13.8244) knots 0 0 0 1 2 2 2
  spline S153 degree 2 poles (5.5275, 13.8244) (5.6807, 13.8244) (6.0465, 13.9035) (6.1701, 14.032) knots 0 0 0 1 2 2 2
  spline S154 degree 2 poles (6.1701, 14.032) (6.264, 14.1358) (6.3827, 14.4374) (6.3827, 14.7092) knots 0 0 0 1 2 2 2
  spline S155 degree 2 poles (6.3827, 14.7092) (6.3827, 14.9811) (6.2146, 15.2728) (6.0811, 15.342) knots 0 0 0 1 2 2 2
  spline S156 degree 2 poles (6.0811, 15.342) (5.9427, 15.4112) (5.5571, 15.426) (5.4138, 15.426) knots 0 0 0 1 2 2 2
  line L247 (5.4138, 15.426) -> (5.2309, 15.426)
  line L248 (5.2309, 15.426) -> (5.2309, 16.4987)
  line L249 (5.2309, 16.4987) -> (5.3989, 16.4987)
  spline S157 degree 2 poles (5.3989, 16.4987) (5.5917, 16.4987) (5.913, 16.5481) (6.0267, 16.6223) knots 0 0 0 1 2 2 2
  spline S158 degree 2 poles (6.0267, 16.6223) (6.1404, 16.7014) (6.269, 16.9782) (6.269, 17.2155) knots 0 0 0 1 2 2 2
  spline S159 degree 2 poles (6.269, 17.2155) (6.269, 17.4033) (6.1503, 17.6357) (6.0613, 17.6999) knots 0 0 0 1 2 2 2
  spline S160 degree 2 poles (6.0613, 17.6999) (5.9575, 17.7741) (5.6857, 17.8235) (5.5868, 17.8235) knots 0 0 0 1 2 2 2
  spline S161 degree 2 poles (5.5868, 17.8235) (5.4335, 17.8235) (5.1073, 17.7197) (4.9541, 17.6357) knots 0 0 0 1 2 2 2
  spline S162 degree 2 poles (4.9541, 17.6357) (4.8354, 17.5714) (4.5734, 17.3638) (4.5092, 17.3094) knots 0 0 0 1 2 2 2
  line L250 (4.5092, 17.3094) -> (4.4202, 17.3094)
  line L251 (4.4202, 17.3094) -> (4.4202, 18.6144)
  spline S163 degree 2 poles (4.4202, 18.6144) (4.6377, 18.7479) (5.3841, 19) (5.7746, 19) knots 0 0 0 1 2 2 2
  spline S164 degree 2 poles (5.7746, 19) (6.1553, 19) (6.7089, 18.8122) (6.9066, 18.6293) knots 0 0 0 1 2 2 2
  spline S165 degree 2 poles (6.9066, 18.6293) (7.1241, 18.4365) (7.3417, 17.8433) (7.3417, 17.4725) knots 0 0 0 1 2 2 2
  spline S166 degree 2 poles (7.3417, 17.4725) (7.3417, 16.9485) (6.9215, 16.1675) (6.5804, 16.0538) knots 0 0 0 1 2 2 2
  line L252 (6.5804, 16.0538) -> (6.5804, 15.9945)
  spline S167 degree 2 poles (6.5804, 15.9945) (6.7336, 15.9648) (7.0203, 15.8066) (7.1588, 15.6287) knots 0 0 0 1 2 2 2
  spline S168 degree 2 poles (7.1588, 15.6287) (7.2873, 15.4705) (7.4553, 14.9663) (7.4553, 14.6203) knots 0 0 0 1 2 2 2
  line L253 (3.6441, 2.7764) -> (0.8264, 2.7764)
  line L254 (0.8264, 2.7764) -> (0.8264, 3.8392)
  line L255 (0.8264, 3.8392) -> (1.7261, 3.8392)
  line L256 (1.7261, 3.8392) -> (1.7261, 7.0672)
  line L257 (1.7261, 7.0672) -> (0.8264, 7.0672)
  line L258 (0.8264, 7.0672) -> (0.8264, 8.0608)
  spline S169 degree 2 poles (0.8264, 8.0608) (1.0241, 8.0608) (1.4147, 8.1349) (1.5333, 8.214) knots 0 0 0 1 2 2 2
  spline S170 degree 2 poles (1.5333, 8.214) (1.6668, 8.3129) (1.82, 8.6441) (1.8299, 8.8912) knots 0 0 0 1 2 2 2
  line L259 (1.8299, 8.8912) -> (2.7642, 8.8912)
  line L260 (2.7642, 8.8912) -> (2.7642, 3.8392)
  line L261 (2.7642, 3.8392) -> (3.6441, 3.8392)
  line L262 (3.6441, 3.8392) -> (3.6441, 2.7764)
  spline S171 degree 2 poles (7.4504, 6.1675) (7.4504, 5.3914) (7.1983, 4.0963) (6.9314, 3.6316) knots 0 0 0 1 2 2 2
  spline S172 degree 2 poles (6.9314, 3.6316) (6.6595, 3.162) (5.8438, 2.6578) (5.2506, 2.6578) knots 0 0 0 1 2 2 2
  spline S173 degree 2 poles (5.2506, 2.6578) (5.048, 2.6578) (4.613, 2.7319) (4.5438, 2.7616) knots 0 0 0 1 2 2 2
  line L263 (4.5438, 2.7616) -> (4.5438, 3.9579)
  line L264 (4.5438, 3.9579) -> (4.6278, 3.9579)
  spline S174 degree 2 poles (4.6278, 3.9579) (4.7069, 3.8985) (5.0035, 3.77) (5.2605, 3.77) knots 0 0 0 1 2 2 2
  spline S175 degree 2 poles (5.2605, 3.77) (5.4731, 3.77) (5.8587, 3.9282) (6.002, 4.1012) knots 0 0 0 1 2 2 2
  spline S176 degree 2 poles (6.002, 4.1012) (6.1454, 4.2841) (6.3431, 4.8229) (6.3777, 5.2283) knots 0 0 0 1 2 2 2
  spline S177 degree 2 poles (6.3777, 5.2283) (6.1454, 5.0256) (5.7549, 4.8081) (5.4632, 4.8081) knots 0 0 0 1 2 2 2
  spline S178 degree 2 poles (5.4632, 4.8081) (5.2408, 4.8081) (4.8354, 4.9762) (4.6723, 5.1541) knots 0 0 0 1 2 2 2
  spline S179 degree 2 poles (4.6723, 5.1541) (4.4498, 5.3964) (4.1928, 6.1724) (4.1928, 6.7854) knots 0 0 0 1 2 2 2
  spline S180 degree 2 poles (4.1928, 6.7854) (4.1928, 7.2649) (4.4202, 8.0707) (4.6278, 8.3673) knots 0 0 0 1 2 2 2
  spline S181 degree 2 poles (4.6278, 8.3673) (4.8354, 8.6639) (5.4335, 9) (5.8043, 9) knots 0 0 0 1 2 2 2
  spline S182 degree 2 poles (5.8043, 9) (6.175, 9) (6.7534, 8.7034) (6.961, 8.392) knots 0 0 0 1 2 2 2
  spline S183 degree 2 poles (6.961, 8.392) (7.2032, 8.0459) (7.4504, 6.9485) (7.4504, 6.1675) knots 0 0 0 1 2 2 2
  spline S184 degree 2 poles (6.3925, 6.3949) (6.3925, 6.8942) (6.2739, 7.5368) (6.1701, 7.7147) knots 0 0 0 1 2 2 2
  spline S185 degree 2 poles (6.1701, 7.7147) (6.0959, 7.8482) (5.9081, 7.9619) (5.7994, 7.9619) knots 0 0 0 1 2 2 2
  spline S186 degree 2 poles (5.7994, 7.9619) (5.7054, 7.9619) (5.5275, 7.8532) (5.4434, 7.7147) knots 0 0 0 1 2 2 2
  spline S187 degree 2 poles (5.4434, 7.7147) (5.3693, 7.5961) (5.2655, 7.1364) (5.2655, 6.8645) knots 0 0 0 1 2 2 2
  spline S188 degree 2 poles (5.2655, 6.8645) (5.2655, 6.5679) (5.3693, 6.1873) (5.4632, 6.0736) knots 0 0 0 1 2 2 2
  spline S189 degree 2 poles (5.4632, 6.0736) (5.5522, 5.9599) (5.7895, 5.8709) (5.9328, 5.8709) knots 0 0 0 1 2 2 2
  spline S190 degree 2 poles (5.9328, 5.8709) (6.0515, 5.8709) (6.3085, 5.9648) (6.3827, 6.0143) knots 0 0 0 1 2 2 2
  spline S191 degree 2 poles (6.3827, 6.0143) (6.3827, 6.0588) (6.3925, 6.2268) (6.3925, 6.3949) knots 0 0 0 1 2 2 2
  line L265 (3.8319, -7.2186) -> (0.6979, -7.2186)
  line L266 (0.6979, -7.2186) -> (0.6979, -6.225)
  spline S192 degree 2 poles (0.6979, -6.225) (1.0983, -5.7703) (1.7261, -4.9694) (1.9683, -4.6086) knots 0 0 0 1 2 2 2
  spline S193 degree 2 poles (1.9683, -4.6086) (2.2797, -4.139) (2.5615, -3.4222) (2.5615, -3.0465) knots 0 0 0 1 2 2 2
  spline S194 degree 2 poles (2.5615, -3.0465) (2.5615, -2.6214) (2.2056, -2.1666) (1.8892, -2.1666) knots 0 0 0 1 2 2 2
  spline S195 degree 2 poles (1.8892, -2.1666) (1.7261, -2.1666) (1.4394, -2.2803) (1.2861, -2.3693) knots 0 0 0 1 2 2 2
  spline S196 degree 2 poles (1.2861, -2.3693) (1.1428, -2.4632) (0.9352, -2.6609) (0.8857, -2.7104) knots 0 0 0 1 2 2 2
  line L267 (0.8857, -2.7104) -> (0.8017, -2.7104)
  line L268 (0.8017, -2.7104) -> (0.8017, -1.3806)
  spline S197 degree 2 poles (0.8017, -1.3806) (0.9797, -1.257) (1.7508, -1) (2.1018, -1) knots 0 0 0 1 2 2 2
  spline S198 degree 2 poles (2.1018, -1) (2.863, -1) (3.6441, -1.9689) (3.6441, -2.8438) knots 0 0 0 1 2 2 2
  spline S199 degree 2 poles (3.6441, -2.8438) (3.6441, -3.3827) (3.2882, -4.4207) (2.8779, -5.0139) knots 0 0 0 1 2 2 2
  spline S200 degree 2 poles (2.8779, -5.0139) (2.6208, -5.3797) (2.1314, -5.9482) (2.0227, -6.0669) knots 0 0 0 1 2 2 2
  line L269 (2.0227, -6.0669) -> (3.8319, -6.0669)
  line L270 (3.8319, -6.0669) -> (3.8319, -7.2186)
  spline S201 degree 2 poles (7.4652, -5.1523) (7.4652, -5.6318) (7.2378, -6.4425) (7.0154, -6.7342) knots 0 0 0 1 2 2 2
  spline S202 degree 2 poles (7.0154, -6.7342) (6.7929, -7.0259) (6.175, -7.3472) (5.7252, -7.3472) knots 0 0 0 1 2 2 2
  spline S203 degree 2 poles (5.7252, -7.3472) (5.2506, -7.3422) (4.5685, -7.1198) (4.346, -6.9764) knots 0 0 0 1 2 2 2
  line L271 (4.346, -6.9764) -> (4.346, -5.6467)
  line L272 (4.346, -5.6467) -> (4.4449, -5.6467)
  spline S204 degree 2 poles (4.4449, -5.6467) (4.524, -5.7109) (4.7217, -5.879) (4.8848, -5.968) knots 0 0 0 1 2 2 2
  spline S205 degree 2 poles (4.8848, -5.968) (5.0381, -6.052) (5.3495, -6.1657) (5.5423, -6.1657) knots 0 0 0 1 2 2 2
  spline S206 degree 2 poles (5.5423, -6.1657) (5.7104, -6.1657) (6.091, -6.0471) (6.2096, -5.8889) knots 0 0 0 1 2 2 2
  spline S207 degree 2 poles (6.2096, -5.8889) (6.2937, -5.7653) (6.3925, -5.4638) (6.3925, -5.2117) knots 0 0 0 1 2 2 2
  spline S208 degree 2 poles (6.3925, -5.2117) (6.3925, -4.9942) (6.269, -4.6877) (6.1701, -4.5938) knots 0 0 0 1 2 2 2
  spline S209 degree 2 poles (6.1701, -4.5938) (6.0218, -4.4553) (5.6115, -4.3763) (5.4632, -4.3763) knots 0 0 0 1 2 2 2
  spline S210 degree 2 poles (5.4632, -4.3763) (5.2259, -4.3763) (4.786, -4.485) (4.6229, -4.5443) knots 0 0 0 1 2 2 2
  line L273 (4.6229, -4.5443) -> (4.5289, -4.5443)
  line L274 (4.5289, -4.5443) -> (4.5289, -1.1186)
  line L275 (4.5289, -1.1186) -> (7.3466, -1.1186)
  line L276 (7.3466, -1.1186) -> (7.3466, -2.2704)
  line L277 (7.3466, -2.2704) -> (5.5374, -2.2704)
  line L278 (5.5374, -2.2704) -> (5.5374, -3.2838)
  spline S211 degree 2 poles (5.5374, -3.2838) (5.6214, -3.2739) (5.8587, -3.264) (5.9279, -3.264) knots 0 0 0 1 2 2 2
  spline S212 degree 2 poles (5.9279, -3.264) (6.2344, -3.264) (6.7534, -3.442) (6.9511, -3.6249) knots 0 0 0 1 2 2 2
  spline S213 degree 2 poles (6.9511, -3.6249) (7.1983, -3.8523) (7.4652, -4.6086) (7.4652, -5.1523) knots 0 0 0 1 2 2 2
  spline S214 degree 2 poles (13.7776, 25.8116) (13.7776, 25.0207) (13.5996, 23.8343) (13.4068, 23.4339) knots 0 0 0 1 2 2 2
  spline S215 degree 2 poles (13.4068, 23.4339) (13.2091, 23.0384) (12.5862, 22.6331) (12.1364, 22.6331) knots 0 0 0 1 2 2 2
  spline S216 degree 2 poles (12.1364, 22.6331) (11.6865, 22.6331) (11.0588, 23.0384) (10.861, 23.4438) knots 0 0 0 1 2 2 2
  spline S217 degree 2 poles (10.861, 23.4438) (10.6682, 23.8442) (10.4903, 25.0207) (10.4903, 25.8116) knots 0 0 0 1 2 2 2
  spline S218 degree 2 poles (10.4903, 25.8116) (10.4903, 26.6223) (10.6633, 27.7691) (10.866, 28.1844) knots 0 0 0 1 2 2 2
  spline S219 degree 2 poles (10.866, 28.1844) (11.0686, 28.5897) (11.6964, 28.9852) (12.1364, 28.9852) knots 0 0 0 1 2 2 2
  spline S220 degree 2 poles (12.1364, 28.9852) (12.5961, 28.9852) (13.2091, 28.5699) (13.4068, 28.1596) knots 0 0 0 1 2 2 2
  spline S221 degree 2 poles (13.4068, 28.1596) (13.6045, 27.7592) (13.7776, 26.5778) (13.7776, 25.8116) knots 0 0 0 1 2 2 2
  spline S222 degree 2 poles (12.7049, 25.8116) (12.7049, 26.9436) (12.4429, 27.8581) (12.1364, 27.8581) knots 0 0 0 1 2 2 2
  spline S223 degree 2 poles (12.1364, 27.8581) (11.825, 27.8581) (11.563, 26.9436) (11.563, 25.8066) knots 0 0 0 1 2 2 2
  spline S224 degree 2 poles (11.563, 25.8066) (11.563, 24.6895) (11.825, 23.7601) (12.1364, 23.7601) knots 0 0 0 1 2 2 2
  spline S225 degree 2 poles (12.1364, 23.7601) (12.4429, 23.7601) (12.7049, 24.6895) (12.7049, 25.8116) knots 0 0 0 1 2 2 2
  spline S226 degree 2 poles (17.5542, 24.4571) (17.5542, 24.0666) (17.3268, 23.3894) (17.1093, 23.1422) knots 0 0 0 1 2 2 2
  spline S227 degree 2 poles (17.1093, 23.1422) (16.8918, 22.8951) (16.264, 22.6182) (15.8587, 22.6182) knots 0 0 0 1 2 2 2
  spline S228 degree 2 poles (15.8587, 22.6182) (15.4286, 22.6182) (14.781, 22.9) (14.5784, 23.1422) knots 0 0 0 1 2 2 2
  spline S229 degree 2 poles (14.5784, 23.1422) (14.3707, 23.3844) (14.178, 24.0419) (14.178, 24.4077) knots 0 0 0 1 2 2 2
  spline S230 degree 2 poles (14.178, 24.4077) (14.178, 24.9317) (14.5833, 25.6287) (14.9639, 25.861) knots 0 0 0 1 2 2 2
  line L279 (14.9639, 25.861) -> (14.9639, 25.8857)
  spline S231 degree 2 poles (14.9639, 25.8857) (14.5882, 26.1477) (14.2917, 26.8942) (14.2917, 27.3539) knots 0 0 0 1 2 2 2
  spline S232 degree 2 poles (14.2917, 27.3539) (14.2917, 27.69) (14.4993, 28.2783) (14.7069, 28.5106) knots 0 0 0 1 2 2 2
  spline S233 degree 2 poles (14.7069, 28.5106) (14.8997, 28.7331) (15.4978, 29) (15.8735, 29) knots 0 0 0 1 2 2 2
  spline S234 degree 2 poles (15.8735, 29) (16.269, 29) (16.8572, 28.7578) (17.0451, 28.56) knots 0 0 0 1 2 2 2
  spline S235 degree 2 poles (17.0451, 28.56) (17.2378, 28.3623) (17.4455, 27.7889) (17.4455, 27.4577) knots 0 0 0 1 2 2 2
  spline S236 degree 2 poles (17.4455, 27.4577) (17.4455, 27.0227) (17.0945, 26.3257) (16.7287, 26.0835) knots 0 0 0 1 2 2 2
  line L280 (16.7287, 26.0835) -> (16.7287, 26.0637)
  spline S237 degree 2 poles (16.7287, 26.0637) (17.1538, 25.8165) (17.5542, 25.0157) (17.5542, 24.4571) knots 0 0 0 1 2 2 2
  spline S238 degree 2 poles (16.4964, 24.3929) (16.4964, 24.6944) (16.3184, 25.0108) (16.0218, 25.2135) knots 0 0 0 1 2 2 2
  spline S239 degree 2 poles (16.0218, 25.2135) (15.9378, 25.2678) (15.6263, 25.4408) (15.5028, 25.515) knots 0 0 0 1 2 2 2
  spline S240 degree 2 poles (15.5028, 25.515) (15.394, 25.3568) (15.216, 24.8823) (15.216, 24.6005) knots 0 0 0 1 2 2 2
  spline S241 degree 2 poles (15.216, 24.6005) (15.216, 24.1754) (15.5967, 23.6662) (15.9081, 23.6662) knots 0 0 0 1 2 2 2
  spline S242 degree 2 poles (15.9081, 23.6662) (15.9921, 23.6662) (16.2096, 23.7453) (16.2937, 23.8244) knots 0 0 0 1 2 2 2
  spline S243 degree 2 poles (16.2937, 23.8244) (16.3827, 23.9183) (16.4964, 24.1754) (16.4964, 24.3929) knots 0 0 0 1 2 2 2
  spline S244 degree 2 poles (16.4074, 27.2797) (16.4074, 27.5912) (16.1207, 27.9619) (15.8735, 27.9619) knots 0 0 0 1 2 2 2
  spline S245 degree 2 poles (15.8735, 27.9619) (15.6412, 27.9619) (15.3495, 27.6258) (15.3495, 27.3786) knots 0 0 0 1 2 2 2
  spline S246 degree 2 poles (15.3495, 27.3786) (15.3495, 27.1364) (15.5225, 26.8348) (15.7104, 26.7113) knots 0 0 0 1 2 2 2
  spline S247 degree 2 poles (15.7104, 26.7113) (15.7895, 26.6519) (16.007, 26.5284) (16.1948, 26.4295) knots 0 0 0 1 2 2 2
  spline S248 degree 2 poles (16.1948, 26.4295) (16.3036, 26.6371) (16.4074, 27.0276) (16.4074, 27.2797) knots 0 0 0 1 2 2 2
  spline S249 degree 2 poles (53.7232, -5.3797) (53.7232, -5.8296) (53.4908, -6.5661) (53.2684, -6.8232) knots 0 0 0 1 2 2 2
  spline S250 degree 2 poles (53.2684, -6.8232) (53.041, -7.0802) (52.433, -7.3571) (51.998, -7.3571) knots 0 0 0 1 2 2 2
  spline S251 degree 2 poles (51.998, -7.3571) (51.4987, -7.3571) (50.7869, -7.1198) (50.5644, -6.9715) knots 0 0 0 1 2 2 2
  line L281 (50.5644, -6.9715) -> (50.5644, -5.6467)
  line L282 (50.5644, -5.6467) -> (50.6682, -5.6467)
  spline S252 degree 2 poles (50.6682, -5.6467) (50.9006, -5.8592) (51.5333, -6.1756) (51.7953, -6.1756) knots 0 0 0 1 2 2 2
  spline S253 degree 2 poles (51.7953, -6.1756) (51.9485, -6.1756) (52.3143, -6.0965) (52.4379, -5.968) knots 0 0 0 1 2 2 2
  spline S254 degree 2 poles (52.4379, -5.968) (52.5318, -5.8642) (52.6505, -5.5626) (52.6505, -5.2908) knots 0 0 0 1 2 2 2
  spline S255 degree 2 poles (52.6505, -5.2908) (52.6505, -5.0189) (52.4824, -4.7272) (52.3489, -4.658) knots 0 0 0 1 2 2 2
  spline S256 degree 2 poles (52.3489, -4.658) (52.2105, -4.5888) (51.825, -4.574) (51.6816, -4.574) knots 0 0 0 1 2 2 2
  line L283 (51.6816, -4.574) -> (51.4987, -4.574)
  line L284 (51.4987, -4.574) -> (51.4987, -3.5013)
  line L285 (51.4987, -3.5013) -> (51.6668, -3.5013)
  spline S257 degree 2 poles (51.6668, -3.5013) (51.8596, -3.5013) (52.1809, -3.4519) (52.2946, -3.3777) knots 0 0 0 1 2 2 2
  spline S258 degree 2 poles (52.2946, -3.3777) (52.4083, -3.2986) (52.5368, -3.0218) (52.5368, -2.7845) knots 0 0 0 1 2 2 2
  spline S259 degree 2 poles (52.5368, -2.7845) (52.5368, -2.5967) (52.4182, -2.3643) (52.3292, -2.3001) knots 0 0 0 1 2 2 2
  spline S260 degree 2 poles (52.3292, -2.3001) (52.2254, -2.2259) (51.9535, -2.1765) (51.8546, -2.1765) knots 0 0 0 1 2 2 2
  spline S261 degree 2 poles (51.8546, -2.1765) (51.7014, -2.1765) (51.3751, -2.2803) (51.2219, -2.3643) knots 0 0 0 1 2 2 2
  spline S262 degree 2 poles (51.2219, -2.3643) (51.1032, -2.4286) (50.8412, -2.6362) (50.777, -2.6906) knots 0 0 0 1 2 2 2
  line L286 (50.777, -2.6906) -> (50.688, -2.6906)
  line L287 (50.688, -2.6906) -> (50.688, -1.3856)
  spline S263 degree 2 poles (50.688, -1.3856) (50.9055, -1.2521) (51.6519, -1) (52.0425, -1) knots 0 0 0 1 2 2 2
  spline S264 degree 2 poles (52.0425, -1) (52.4231, -1) (52.9767, -1.1878) (53.1745, -1.3707) knots 0 0 0 1 2 2 2
  spline S265 degree 2 poles (53.1745, -1.3707) (53.392, -1.5635) (53.6095, -2.1567) (53.6095, -2.5275) knots 0 0 0 1 2 2 2
  spline S266 degree 2 poles (53.6095, -2.5275) (53.6095, -3.0515) (53.1893, -3.8325) (52.8482, -3.9462) knots 0 0 0 1 2 2 2
  line L288 (52.8482, -3.9462) -> (52.8482, -4.0055)
  spline S267 degree 2 poles (52.8482, -4.0055) (53.0015, -4.0352) (53.2882, -4.1934) (53.4266, -4.3713) knots 0 0 0 1 2 2 2
  spline S268 degree 2 poles (53.4266, -4.3713) (53.5551, -4.5295) (53.7232, -5.0337) (53.7232, -5.3797) knots 0 0 0 1 2 2 2
  spline S269 degree 2 poles (57.5097, -4.1785) (57.5097, -4.9694) (57.3318, -6.1558) (57.139, -6.5562) knots 0 0 0 1 2 2 2
  spline S270 degree 2 poles (57.139, -6.5562) (56.9412, -6.9517) (56.3184, -7.3571) (55.8686, -7.3571) knots 0 0 0 1 2 2 2
  spline S271 degree 2 poles (55.8686, -7.3571) (55.4187, -7.3571) (54.7909, -6.9517) (54.5932, -6.5464) knots 0 0 0 1 2 2 2
  spline S272 degree 2 poles (54.5932, -6.5464) (54.4004, -6.1459) (54.2224, -4.9694) (54.2224, -4.1785) knots 0 0 0 1 2 2 2
  spline S273 degree 2 poles (54.2224, -4.1785) (54.2224, -3.3678) (54.3955, -2.221) (54.5981, -1.8058) knots 0 0 0 1 2 2 2
  spline S274 degree 2 poles (54.5981, -1.8058) (54.8008, -1.4004) (55.4286, -1.0049) (55.8686, -1.0049) knots 0 0 0 1 2 2 2
  spline S275 degree 2 poles (55.8686, -1.0049) (56.3283, -1.0049) (56.9412, -1.4202) (57.139, -1.8305) knots 0 0 0 1 2 2 2
  spline S276 degree 2 poles (57.139, -1.8305) (57.3367, -2.2309) (57.5097, -3.4123) (57.5097, -4.1785) knots 0 0 0 1 2 2 2
  spline S277 degree 2 poles (56.437, -4.1785) (56.437, -3.0465) (56.175, -2.132) (55.8686, -2.132) knots 0 0 0 1 2 2 2
  spline S278 degree 2 poles (55.8686, -2.132) (55.5571, -2.132) (55.2951, -3.0465) (55.2951, -4.1835) knots 0 0 0 1 2 2 2
  spline S279 degree 2 poles (55.2951, -4.1835) (55.2951, -5.3006) (55.5571, -6.23) (55.8686, -6.23) knots 0 0 0 1 2 2 2
  spline S280 degree 2 poles (55.8686, -6.23) (56.175, -6.23) (56.437, -5.3006) (56.437, -4.1785) knots 0 0 0 1 2 2 2
  line L289 (43.8319, -7.2236) -> (40.6979, -7.2236)
  line L290 (40.6979, -7.2236) -> (40.6979, -6.23)
  spline S281 degree 2 poles (40.6979, -6.23) (41.0983, -5.7752) (41.7261, -4.9744) (41.9683, -4.6135) knots 0 0 0 1 2 2 2
  spline S282 degree 2 poles (41.9683, -4.6135) (42.2797, -4.1439) (42.5615, -3.4271) (42.5615, -3.0515) knots 0 0 0 1 2 2 2
  spline S283 degree 2 poles (42.5615, -3.0515) (42.5615, -2.6263) (42.2056, -2.1716) (41.8892, -2.1716) knots 0 0 0 1 2 2 2
  spline S284 degree 2 poles (41.8892, -2.1716) (41.7261, -2.1716) (41.4394, -2.2853) (41.2861, -2.3742) knots 0 0 0 1 2 2 2
  spline S285 degree 2 poles (41.2861, -2.3742) (41.1428, -2.4682) (40.9352, -2.6659) (40.8857, -2.7153) knots 0 0 0 1 2 2 2
  line L291 (40.8857, -2.7153) -> (40.8017, -2.7153)
  line L292 (40.8017, -2.7153) -> (40.8017, -1.3856)
  spline S286 degree 2 poles (40.8017, -1.3856) (40.9797, -1.262) (41.7508, -1.0049) (42.1018, -1.0049) knots 0 0 0 1 2 2 2
  spline S287 degree 2 poles (42.1018, -1.0049) (42.863, -1.0049) (43.6441, -1.9738) (43.6441, -2.8488) knots 0 0 0 1 2 2 2
  spline S288 degree 2 poles (43.6441, -2.8488) (43.6441, -3.3876) (43.2882, -4.4257) (42.8779, -5.0189) knots 0 0 0 1 2 2 2
  spline S289 degree 2 poles (42.8779, -5.0189) (42.6208, -5.3847) (42.1314, -5.9532) (42.0227, -6.0718) knots 0 0 0 1 2 2 2
  line L293 (42.0227, -6.0718) -> (43.8319, -6.0718)
  line L294 (43.8319, -6.0718) -> (43.8319, -7.2236)